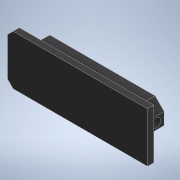
# Autodesk Inventor part: Magazin_Stössel
Saved by Autodesk Inventor 2021 (Build 250183000, 183)
## iProperties
Created: 2024-05-14
Part Number: Magazin_Stössel
Material: Generic
Document SubType Name: Modeling
Designer: Lukas
Density: 1 g/cm^3
Appearance: Default
Author: Lukas
Autodesk Inventor part; units mm, degrees
ref_plane "YZ Plane" through (0, 0, 0) normal (1, 0, 0) x (0, 1, 0)
ref_plane "XZ Plane" through (0, 0, 0) normal (0, 1, 0) x (-1, 0, 0)
ref_plane "XY Plane" through (0, 0, 0) normal (0, 0, 1) x (1, 0, 0)
sketch "Sketch1" plane through (0, 0, 0) normal (0, 0, 1) x (1, 0, 0)
  line L0 (-20, 2) -> (-17, 5)
  line L1 (-17, 5) -> (17, 5)
  line L2 (17, 5) -> (20, 2)
  line L3 (20, 2) -> (20, -2)
  line L4 (20, -2) -> (17, -5)
  line L5 (17, -5) -> (-17, -5)
  line L6 (-17, -5) -> (-20, -2)
  line L7 (-20, -2) -> (-20, 2)
  line L8 (16.9379, 4.85) -> (-16.9379, 4.85)
  line L9 (-16.9379, 4.85) -> (-19.85, 1.9379)
  line L10 (-19.85, 1.9379) -> (-19.85, -1.9379)
  line L11 (-19.85, -1.9379) -> (-16.9379, -4.85)
  line L12 (-16.9379, -4.85) -> (16.9379, -4.85)
  line L13 (16.9379, -4.85) -> (19.85, -1.9379)
  line L14 (19.85, -1.9379) -> (19.85, 1.9379)
  line L15 (19.85, 1.9379) -> (16.9379, 4.85)
  point P0 (0, 0)
  point P1 (0, 5)
  point P2 (-20, 0)
  dimension "d0" = 3
  dimension "d1" = 3
  dimension "d2" = 10
  dimension "d3" = 34
  dimension "d4" = 0.15
  constraints: 32 end point, 9 perpendicular, 4 parallel, 2 midpoint, 2 vertical alignment, 1 horizontal, 1 horizontal alignment, 7 other
  measures "d0" horizontal distance of L0.start L0.end
  measures "d1" horizontal distance of L0.start L0.end
  measures "d2" distance between parallel lines of L5 L1
  measures "d3" distance of L0.end L1.end
  measures "d4" distance between parallel lines of L1 L8
extrude "Extrusion1" add sketch "Sketch1" along normal blind 6 contours L15 L14 L13 L12 L11 L10 L9 L8
sketch "Sketch4" plane through (0, 0, 6) normal (0, 0, 1) x (1, 0, 0)
  line L0 (-16.9379, 4.85) -> (-19.85, 1.9379) projected
  line L1 (-19.85, 1.9379) -> (-19.85, -1.9379) projected
  line L2 (-19.85, -1.9379) -> (-16.9379, -4.85) projected
  line L3 (-16.9379, -4.85) -> (16.9379, -4.85) projected
  line L4 (16.9379, -4.85) -> (19.85, -1.9379) projected
  line L5 (19.85, -1.9379) -> (19.85, 1.9379) projected
  line L6 (19.85, 1.9379) -> (16.9379, 4.85) projected
  line L7 (16.9379, 4.85) -> (-16.9379, 4.85) projected
  line L8 (22.5, -8) -> (22.5, 8)
  line L9 (22.5, 8) -> (-20.7, 8)
  line L10 (-20.7, 8) -> (-22.5, 6.2)
  line L11 (-22.5, 6.2) -> (-22.5, -6.2)
  line L12 (-22.5, -6.2) -> (-20.7, -8)
  line L13 (-20.7, -8) -> (22.5, -8)
  point P0 (0, 0)
  point P1 (22.5, 0)
  dimension "d20" = 45
  dimension "d21" = 16
  dimension "d22" = 1.8
  dimension "d23" = 1.8
  dimension "d24" = 1.8
  dimension "d25" = 22.5
  constraints: 12 end point, 2 perpendicular, 1 horizontal, 1 horizontal alignment, 1 midpoint, 1 parallel, 1 vertical
  measures "d20" distance between parallel lines of L8 L11
  measures "d21" distance of L8.start L8.end
  measures "d22" horizontal distance of L9.end L10.end
  measures "d23" horizontal distance of L9.end L10.end
  measures "d24" horizontal distance of L11.end L12.end
  measures "d25" distance from line of point (0, 0) L11
extrude "Extrusion4" add sketch "Sketch4" along normal blind 2 contours L7 L6 L5 L4 L3 L2 L1 L0 | L13 L12 L11 L10 L9 L8
sketch "Sketch5" plane through (-19.85, -1.9379, 0) normal (-1, 0, 0) x (0, 0, 1)
  circle A0 centre (2.5, 1.9379) radius 1.4
  line L0 (0, 3.8757) -> (0, 0) projected
  line L1 (6, 3.8757) -> (6, 0) projected
  point P0 (0, 1.9379)
  point P1 (0, 1.9379)
  dimension "d28" = 3.5
  dimension "d29" = 2.8
  constraints: 1 centre point, 1 horizontal alignment, 1 midpoint
  measures "d28" distance from line of L1 A0.centre
  measures "d29" diameter of A0
extrude "Extrusion5" cut sketch "Sketch5" against normal blind 8
mirror "Mirror1" about plane through (0, 0, 0) normal (1, 0, 0) of "Extrusion5"
equation "\"d24\" = d23"
equation "\"d25\" = 0.5 * d20"
body "Solid1"
